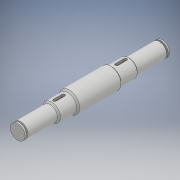
# Autodesk Inventor part: Вал 3
Saved by Autodesk Inventor 2018.1 (Build 221171000, 171)
## iProperties
Created: 2018-06-08
Part Number: Вал 3
Material: Типовые
Document SubType Name: Modeling
Designer: Dmitry
Density: 1 g/cm^3
Appearance: По умолчанию
Author: Dmitry
Autodesk Inventor part; units mm, degrees
ref_plane "YZ Plane" through (0, 0, 0) normal (1, 0, 0) x (0, 1, 0)
ref_plane "XZ Plane" through (0, 0, 0) normal (0, 1, 0) x (-1, 0, 0)
ref_plane "XY Plane" through (0, 0, 0) normal (0, 0, 1) x (1, 0, 0)
sketch "Эскиз1" plane through (0, 0, 0) normal (0, 0, 1) x (1, 0, 0)
  line L0 (0, 0) -> (25, 0)
  line L1 (25, 0) -> (25, 5)
  line L2 (25, 5) -> (20, 5)
  line L3 (20, 5) -> (20, 10)
  line L4 (20, 10) -> (25, 10)
  line L5 (25, 10) -> (25, 110)
  line L6 (25, 110) -> (30, 110)
  line L7 (30, 110) -> (30, 170)
  line L8 (30, 170) -> (35, 170)
  line L9 (35, 170) -> (35, 320)
  line L10 (35, 320) -> (30, 320)
  line L11 (30, 320) -> (30, 380)
  line L12 (30, 380) -> (25, 380)
  line L13 (25, 380) -> (25, 480)
  line L14 (25, 480) -> (20, 480)
  line L15 (20, 480) -> (20, 485)
  line L16 (20, 485) -> (25, 485)
  line L17 (25, 485) -> (25, 490)
  line L18 (25, 490) -> (0, 490)
  line L19 (0, 490) -> (0, 0)
  line L20 (0, -98) -> (0, 588) projected
  constraints: 40 end point
revolve "Вращение1" add sketch "Эскиз1" angle 360 about axis through (0, -10, 0) along (0, 1, 0)
sketch "Эскиз2" plane through (0, 0, 30) normal (0, 0, 1) x (1, 0, 0)
  line L0 (-5, 125) -> (-5, 155)
  line L1 (5, 125) -> (5, 155)
  arc A0 (-5, 125) -> (5, 125) centre (0, 125) ccw
  arc A1 (5, 155) -> (-5, 155) centre (0, 155) ccw
  line L2 (-5, 335) -> (-5, 365)
  line L3 (5, 335) -> (5, 365)
  arc A2 (-5, 335) -> (5, 335) centre (0, 335) ccw
  arc A3 (5, 365) -> (-5, 365) centre (0, 365) ccw
  constraints: 8 end point, 8 point on circle, 4 centre point
extrude "Выдавливание1" cut sketch "Эскиз2" against normal blind 10
sketch "Эскиз3" plane through (0, 0, -25) normal (0, 0, 1) x (1, 0, 0)
  line L0 (5, 125) -> (5, 250)
  line L1 (-5, 125) -> (-5, 250)
  arc A0 (-5, 125) -> (5, 125) centre (0, 125) ccw
  arc A1 (5, 250) -> (-5, 250) centre (0, 250) ccw
  line L2 (5, 40) -> (5, 80)
  line L3 (-5, 40) -> (-5, 80)
  arc A2 (-5, 40) -> (5, 40) centre (0, 40) ccw
  arc A3 (5, 80) -> (-5, 80) centre (0, 80) ccw
  constraints: 8 end point, 8 point on circle, 4 centre point
extrude "Выдавливание2" cut sketch "Эскиз3" along normal blind 10
mirror "Зеркальное отражение1" about plane through (0, 245, 0) normal (0, 1, 0) of "Выдавливание2"
chamfer "Фаска1" distance 5 angle 45 4 edges at (-30, 110, 0) (-35, 170, 0) (-35, 320, 0) (-30, 380, 0)
